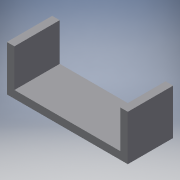
# Autodesk Inventor part: encaje
Saved by Autodesk Inventor 2018 (Build 220112000, 112)
## iProperties
Created: 2021-07-06
Part Number: encaje
Material: Genérico
Document SubType Name: Modeling
Designer: GABRIEL
Density: 1 g/cm^3
Appearance: Valor por defecto
Author: GABRIEL
Autodesk Inventor part; units mm, degrees
ref_plane "YZ Plane" through (0, 0, 0) normal (1, 0, 0) x (0, 1, 0)
ref_plane "XZ Plane" through (0, 0, 0) normal (0, 1, 0) x (-1, 0, 0)
ref_plane "XY Plane" through (0, 0, 0) normal (0, 0, 1) x (1, 0, 0)
sketch "Boceto1" plane through (0, 0, 0) normal (0, 1, 0) x (-1, 0, 0)
  line L0 (0, 0) -> (80, 0)
  line L1 (80, 0) -> (80, 35)
  line L2 (80, 35) -> (0, 35)
  line L3 (0, 35) -> (0, 0)
  line L4 (75, 35) -> (5, 35)
  line L5 (5, 35) -> (5, 5)
  line L6 (5, 5) -> (75, 5)
  line L7 (75, 5) -> (75, 35)
  dimension "d0" = 80
  dimension "d1" = 35
  dimension "d2" = 70
  dimension "d3" = 30
  dimension "d14" = 5
  constraints: 16 end point, 4 parallel, 2 horizontal, 2 perpendicular, 1 point on line
  measures "d0" distance of L2.end L1.end
  measures "d1" distance of L1.end L0.end
  measures "d2" distance of L6.end L5.end
  measures "d3" distance of L5.end L4.end
  measures "d14" distance between parallel lines of L0 L6
extrude "Extrusión1" add sketch "Boceto1" along normal blind 30 contours L3 L2 L5 L6 L7 L1 L0
sketch "Boceto2" plane through (-75, 0, 5) normal (0, 0, 1) x (1, 0, 0)
  circle A0 centre (35, 15) radius 10
  point P0 (75, 0)
  dimension "d6" = 20
  constraints: 1 centre point
  measures "d6" diameter of A0
extrude "Extrusión2" cut sketch "Boceto2" against normal blind 30
sketch "Boceto3" plane through (-75, 0, 5) normal (1, 0, 0) x (0, 0, -1)
  circle A0 centre (-22, 15) radius 2.5
  line L0 (-30, 0) -> (-30, 30) projected
  line L1 (-30, 30) -> (0, 30) projected
  point P0 (5, 0)
  dimension "d9" = 5
  dimension "d12" = 8
  dimension "d13" = 15
  constraints: 1 centre point
  measures "d9" diameter of A0
  measures "d12" distance from line of L0 A0.centre
  measures "d13" distance from line of L1 A0.centre
extrude "Extrusión3" add sketch "Boceto3" along normal blind 70
